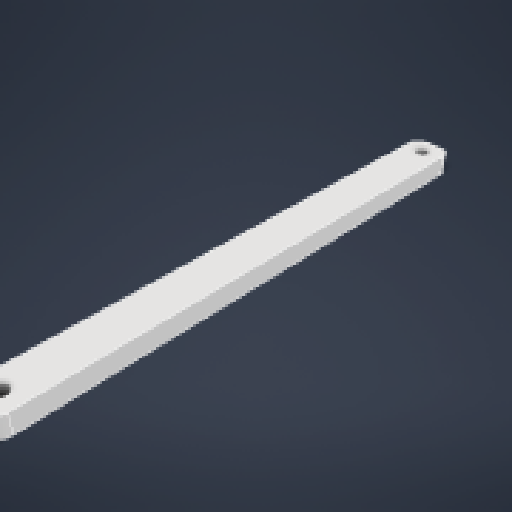
# Autodesk Inventor part: Steering_Linkage
Saved by Autodesk Inventor 2025 (Build 290162000, 162)
## iProperties
Created: 2024-05-24
Part Number: Steering_Linkage
Material: Generic
Document SubType Name: Modeling
Designer: Garfieldcmix
Density: 1 g/cm^3
Appearance: Default
Author: Garfieldcmix
Autodesk Inventor part; units mm, degrees
ref_plane "YZ Plane" through (0, 0, 0) normal (1, 0, 0) x (0, 1, 0)
ref_plane "XZ Plane" through (0, 0, 0) normal (0, 1, 0) x (-1, 0, 0)
ref_plane "XY Plane" through (0, 0, 0) normal (0, 0, 1) x (1, 0, 0)
sketch "Sketch1" plane through (0, 0, 0) normal (0, 1, 0) x (-1, 0, 0)
  line L0 (0, 0) -> (6, 0)
  line L1 (6, 0) -> (6, -82)
  line L2 (6, -82) -> (0, -82)
  line L3 (0, -82) -> (0, 0)
  circle A0 centre (3, -3) radius 1
  circle A1 centre (3, -79) radius 1
  circle A2 centre (3, -41) radius 1
  point P0 (3, 0)
  point P1 (6, -41)
  dimension "d0" = 6
  dimension "d1" = 82
  dimension "d2" = 2
  dimension "d3" = 2
  dimension "d4" = 76
  dimension "d5" = 3
  dimension "d6" = 3
  dimension "d7" = 3
  dimension "d11" = 2
  dimension "d12" = 3
  dimension "d13" = 41
  constraints: 8 end point, 3 centre point, 2 midpoint, 2 parallel, 1 horizontal, 1 perpendicular
  measures "d0" distance of L1.end L2.end
  measures "d1" distance of L0.end L1.end
  measures "d2" diameter of A0
  measures "d3" diameter of A1
  measures "d4" distance of A1.centre A0.centre
  measures "d5" distance of point (3, 0) A0.centre
  measures "d6" distance from line of L1 A0.centre
  measures "d7" distance from line of L1 A1.centre
  measures "d11" diameter of A2
  measures "d12" distance of point (6, -41) A2.centre
  measures "d13" distance from line of L0 A2.centre
extrude "Extrusion1" add sketch "Sketch1" along normal blind 3
fillet "Fillet1" radius 2 4 edges at (0, 1.5, 0) (-6, 1.5, 0) (0, 1.5, -82) (-6, 1.5, -82)
equation "\"d6\" = 0.5 * d0"
equation "\"d7\" = d6"
equation "\"d12\" = 0.5 * d0"
equation "\"d13\" = 0.5 * d1"
body "Solid1"
